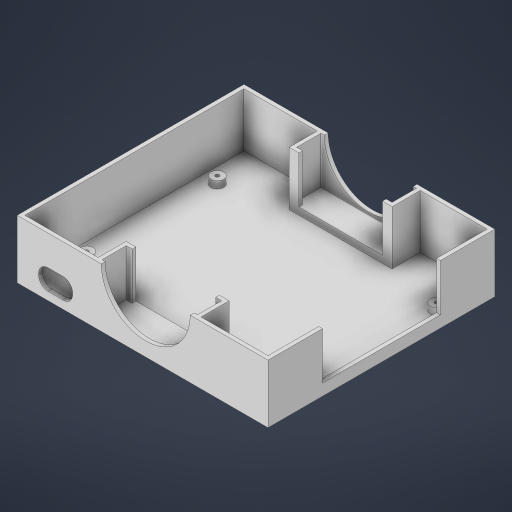
# Autodesk Inventor part: orangepicover-002
Saved by Autodesk Inventor 2023 (Build 270158000, 158)
## iProperties
Created: 2024-02-19
Part Number: orangepicover-002
Material: Generic
Document SubType Name: Modeling
Designer: Paul
Density: 1 g/cm^3
Appearance: Default
Author: Paul
Autodesk Inventor part; units mm, degrees
ref_plane "Work Plane1" through (0, 0, 0) normal (0, 0, 1) x (1, 0, 0)
sketch "Sketch1" plane through (0, 0, 0) normal (0, 0, 1) x (1, 0, 0)
  line L0 (-51.7982, 21.731) -> (-51.7982, 11.231) projected
  line L1 (-52.2736, -10.8209) -> (-52.2736, 4.8763)
  line L2 (4.6436, -33.7466) -> (19.655, -33.7466)
  line L3 (52.2917, 11.1414) -> (52.2917, 22.8908)
  line L4 (53.3077, -47.7466) -> (53.3077, 45.916)
  line L5 (-48.73, 30.9) -> (48.73, 30.9) projected
  line L6 (-52.2736, 31.916) -> (53.3077, 31.916) construction
  line L7 (-50.6226, 45.916) -> (53.3077, 45.916)
  line L8 (-50.6226, -47.7466) -> (53.3077, -47.7466)
  line L9 (-52.2736, 47.567) -> (-52.2736, -49.3976)
  line L10 (-50.6226, 45.916) -> (-50.6226, -47.7466)
  line L11 (54.9587, 47.567) -> (-52.2736, 47.567)
  line L12 (-52.2736, -49.3976) -> (54.9587, -49.3976)
  line L13 (54.9587, -49.3976) -> (54.9587, 47.567)
  point P0 (0, 0)
  dimension "d0" = 1.016
  dimension "d1" = 1.016
  dimension "d2" = 14
  dimension "d3" = 14
  dimension "d5" = 1.651
  dimension "d6" = 1.651
  dimension "d7" = 1.651
  dimension "d8" = 0
  dimension "d9" = 1.651
  constraints: 24 end point, 4 parallel, 2 point on line, 2 vertical, 1 horizontal, 6 other
  measures "d0" distance between parallel lines of L3 L4
  measures "d1" distance between parallel lines of L5 L6
  measures "d2" distance between parallel lines of L6 L7
  measures "d3" distance between parallel lines of L2 L8
  measures "d5" distance between parallel lines of L7 L11
  measures "d6" distance between parallel lines of L12 L8
  measures "d7" distance between parallel lines of L4 L13
  measures "d8" distance between parallel lines of L1 L9
  measures "d9" distance between parallel lines of L9 L10
extrude "Extrusion1" add sketch "Sketch1" against normal blind 20
sketch "Sketch2" plane through (0, 0, 0) normal (0, 0, 1) x (1, 0, 0)
  line L0 (-52.2736, 47.567) -> (-52.2736, -49.3976) projected
  line L1 (-52.2736, -49.3976) -> (54.9587, -49.3976) projected
  line L2 (54.9587, -49.3976) -> (54.9587, 47.567) projected
  line L3 (54.9587, 47.567) -> (-52.2736, 47.567) projected
  line L4 (-50.6226, 45.916) -> (53.3077, 45.916) projected
  line L5 (53.3077, 45.916) -> (53.3077, -47.7466) projected
  line L6 (53.3077, -47.7466) -> (-50.6226, -47.7466) projected
  line L7 (-50.6226, -47.7466) -> (-50.6226, 45.916) projected
  point P0 (0, 0)
extrude "Extrusion2" add sketch "Sketch2" along normal blind 5
sketch "Sketch3" plane through (0, 0, 5) normal (0, 0, 1) x (1, 0, 0)
  line L0 (-52.2736, 47.567) -> (-52.2736, -49.3976) projected
  line L1 (54.9587, 47.567) -> (-52.2736, 47.567) projected
  line L2 (54.9587, -49.3976) -> (54.9587, 47.567) projected
  line L3 (-52.2736, -49.3976) -> (54.9587, -49.3976) projected
  point P0 (0, 0)
extrude "Extrusion3" add sketch "Sketch3" against normal blind 2
sketch "Sketch4" plane through (0, 0, 3) normal (0, 0, -1) x (-1, 0, 0)
  circle A0 centre (47.0077, 28.0411) radius 1.45 construction
  circle A1 centre (-46.8473, 28.0411) radius 1.45 construction
  circle A2 centre (-46.8473, -27.8489) radius 1.45 construction
  circle A3 centre (47.0077, -27.8489) radius 1.45 construction
  circle A4 centre (47.0077, -27.8489) radius 2.72
  circle A5 centre (-46.8473, -27.8489) radius 2.72
  circle A6 centre (-46.8473, 28.0411) radius 2.72
  circle A7 centre (47.0077, 28.0411) radius 2.72
  point P0 (0, 0)
  dimension "d16" = 1.27
  constraints: 4 centre point, 3 equal radius
  measures "d16" radial gap between concentric circles of A3 A4
extrude "Extrusion4" add sketch "Sketch4" along normal blind 3
sketch "Sketch5" plane through (-52.2736, -49.3976, -20) normal (-1, 0, 0) x (0, 0, 1)
  line L0 (17.7, 27.0811) -> (5.5, 27.0811) projected
  line L1 (2.6, 71.1286) -> (2.6, 60.6286) projected
  line L2 (4.16, 72.4286) -> (8.16, 72.4286) projected
  line L3 (18.8, 72.9298) -> (18.8, 19.7676)
  line L4 (18.8, 27.0811) -> (2.6, 27.0811) construction
  line L5 (2.6, 27.0811) -> (2.6, 72.4287) construction
  line L6 (2.6, 72.4287) -> (18.8, 72.4287) construction
  line L7 (18.8, 72.4287) -> (18.8, 27.0811) construction
  line L8 (20.07, 23.2711) -> (20.07, 73.6987)
  line L9 (20.07, 73.6987) -> (0, 73.6987)
  line L10 (20.07, 23.2711) -> (0, 23.2711)
  line L11 (0, 96.9646) -> (0, 73.6935) projected
  line L12 (0, 0) -> (0, 96.9646) projected
  point P0 (20, 49.3976)
  dimension "d19" = 16.2
  dimension "d28" = 45.3475
  dimension "d29" = 1.27
  dimension "d30" = 3.81
  dimension "d31" = 1.27
  constraints: 16 end point, 4 point on line, 2 parallel, 1 horizontal, 1 perpendicular, 1 vertical, 2 other
  measures "d19" distance of L4.start L4.end
  measures "d28" distance of L4.end L5.end
  measures "d29" distance between parallel lines of L9 L2
  measures "d30" distance between parallel lines of L10 L0
  measures "d31" distance between parallel lines of L8 L7
extrude "Extrusion5" cut sketch "Sketch5" against normal blind 3
sketch "Sketch6" plane through (-52.2736, -49.3976, -20) normal (0, -1, 0) x (1, 0, 0)
  spline S0 degree 3 poles (96.7423, 17.4713) (96.7421, 17.4836) (96.7307, 17.9286) (96.5147, 18.8754) (95.3569, 20.0332) (94.4077, 20.2413) (93.9636, 20.25) knots 0 0 0 0 0.009266 0.335677 0.66431 1 1 1 1 construction
  line L0 (93.9636, 20.25) -> (87.581, 20.25) construction
  spline S1 degree 3 poles (87.581, 20.25) (87.5687, 20.2498) (87.1237, 20.2384) (86.1769, 20.0224) (85.0191, 18.8646) (84.811, 17.9154) (84.8023, 17.4713) knots 0 0 0 0 0.009266 0.335677 0.66431 1 1 1 1 construction
  line L1 (84.8023, 17.4713) -> (84.8023, 16.8687) construction
  spline S2 degree 3 poles (84.8023, 16.8687) (84.8025, 16.8564) (84.8139, 16.4114) (85.0299, 15.4646) (86.1877, 14.3068) (87.1369, 14.0987) (87.581, 14.09) knots 0 0 0 0 0.009266 0.335677 0.66431 1 1 1 1 construction
  line L2 (87.581, 14.09) -> (93.9636, 14.09) construction
  spline S3 degree 3 poles (93.9636, 14.09) (93.9759, 14.0902) (94.4209, 14.1016) (95.3677, 14.3176) (96.5255, 15.4754) (96.7336, 16.4246) (96.7423, 16.8687) knots 0 0 0 0 0.009266 0.335677 0.66431 1 1 1 1 construction
  line L3 (96.7423, 16.8687) -> (96.7423, 17.4713) construction
  circle A0 centre (90.7723, 17.17) radius 2.5 construction
  line L4 (93.9884, 12.82) -> (87.5562, 12.82)
  line L5 (83.5323, 16.8439) -> (83.5323, 17.4961)
  line L6 (87.5562, 21.52) -> (93.9884, 21.52)
  line L7 (98.0123, 17.4961) -> (98.0123, 16.8439)
  spline S4 degree 4 poles (87.5562, 12.8202) (87.0451, 12.8307) (86.5365, 12.9185) (85.5165, 13.2808) (84.696, 13.9837) (83.9931, 14.8042) (83.6308, 15.8242) (83.543, 16.3328) (83.5325, 16.8439) knots 0 0 0 0 0 0.32448 0.32448 0.675511 0.675511 1 1 1 1 1
  spline S5 degree 4 poles (83.5325, 17.4961) (83.5431, 18.0072) (83.6308, 18.5158) (83.9931, 19.5358) (84.696, 20.3563) (85.5165, 21.0592) (86.5365, 21.4215) (87.0451, 21.5092) (87.5562, 21.5198) knots 0 0 0 0 0 0.32448 0.32448 0.675511 0.675511 1 1 1 1 1
  spline S6 degree 4 poles (93.9884, 21.5198) (94.4995, 21.5092) (95.0081, 21.4215) (96.0281, 21.0592) (96.8486, 20.3563) (97.5515, 19.5358) (97.9138, 18.5158) (98.0016, 18.0072) (98.0121, 17.4961) knots 0 0 0 0 0 0.32448 0.32448 0.675511 0.675511 1 1 1 1 1
  spline S7 degree 4 poles (98.0121, 16.8439) (98.0015, 16.3328) (97.9138, 15.8242) (97.5515, 14.8042) (96.8486, 13.9837) (96.0281, 13.2808) (95.0081, 12.9185) (94.4995, 12.8307) (93.9884, 12.8202) knots 0 0 0 0 0 0.32448 0.32448 0.675511 0.675511 1 1 1 1 1
  point P0 (52.2736, 20)
  dimension "d24" = 1.27
  constraints: 8 end point, 7 parallel, 12 other
  measures "d24" distance between parallel lines of L2 L4
extrude "Extrusion6" cut sketch "Sketch6" against normal blind 3
sketch "Sketch7" plane through (0, 0, 3) normal (0, 0, -1) x (-1, 0, 0)
  line L0 (50.6226, -47.7466) -> (-53.3077, -47.7466) projected
  line L1 (0, -68.7905) -> (0, 66.9599) projected
  line L2 (50.6226, -47.7466) -> (-53.3077, -47.7466) projected
  line L3 (-22, -47.7466) -> (22, -47.7466)
  line L4 (22, -47.7466) -> (22, -35.7466)
  line L5 (22, -35.7466) -> (-22, -35.7466)
  line L6 (-22, -35.7466) -> (-22, -47.7466)
  point P0 (0, 0)
  point P1 (22, -47.7466)
  dimension "d32" = 44
  dimension "d33" = 22
  dimension "d34" = 12
  constraints: 8 end point, 2 parallel, 1 horizontal, 1 perpendicular, 1 point on line
  measures "d32" distance of L4.end L5.end
  measures "d33" distance between parallel lines of L6 L1
  measures "d34" distance of L3.end L4.end
ref_plane "Work Plane2" through (-18.0279, -47.6958, 0.0279) normal (0, 0, 1) x (1, 0, 0)
extrude "Extrusion7" add sketch "Sketch7" along normal up to surface (2.9721 mm away)
sketch "Sketch8" plane through (22, -35.7466, 0.0279) normal (0, 0, -1) x (-1, 0, 0)
  line L0 (44, 0) -> (0, 0) projected
  line L1 (0, 0) -> (0, -12) projected
  line L2 (44, -12) -> (0, -12) construction
  line L3 (44, -12) -> (44, 0) projected
  line L4 (42.4, -1.6) -> (42.4, -12)
  line L5 (1.6, -12) -> (1.6, -1.6)
  line L6 (4.14, 0) -> (4.14, -1.6)
  line L7 (1.6, -1.6) -> (4.14, -1.6)
  line L8 (39.86, -1.6) -> (42.4, -1.6)
  line L9 (0, -12) -> (1.6, -12)
  line L10 (42.4, -12) -> (44, -12)
  line L11 (39.86, -1.6) -> (39.86, 0)
  point P0 (22, 35.7466)
  point P1 (4.14, -0.8)
  dimension "d47" = 2.54
  dimension "d48" = 2.54
  dimension "d49" = 1.6
  dimension "d50" = 1.6
  dimension "d51" = 1.6
  dimension "d52" = 1.6
  constraints: 16 end point, 4 point on line, 3 perpendicular, 2 collinear, 1 midpoint
  measures "d47" distance from line of L5 point (4.14, -0.8)
  measures "d48" distance between parallel lines of L4 L11
  measures "d49" distance between parallel lines of L1 L5
  measures "d50" distance between parallel lines of L0 L7
  measures "d51" distance between parallel lines of L3 L4
  measures "d52" distance between parallel lines of L0 L8
extrude "Extrusion8" add sketch "Sketch8" along normal up to surface (20.0279 mm away)
sketch "Sketch9" plane through (-52.2736, -49.3976, -20) normal (0, -1, 0) x (1, 0, 0)
  line L0 (52.2736, 30) -> (52.2736, -5) projected
  line L1 (107.2323, 0) -> (0, 0) projected
  arc A0 (71.2736, 0) -> (33.2736, 0) centre (52.2736, 0) ccw
  point P0 (52.2736, 20)
  dimension "d53" = 38
  constraints: 4 point on line, 2 point on circle, 1 centre point
  measures "d53" diameter of A0
extrude "Extrusion9" cut sketch "Sketch9" against normal up to surface (1.651 mm away)
sketch "Sketch10" plane through (0, 0, 3) normal (0, 0, -1) x (-1, 0, 0)
  line L0 (0, -68.7905) -> (0, 66.9599) construction
  line L1 (-53.3077, 45.916) -> (50.6226, 45.916) construction
  line L2 (22, 45.916) -> (-22, 45.916)
  line L3 (-22, 45.916) -> (-22, 33.916)
  line L4 (-22, 33.916) -> (22, 33.916)
  line L5 (22, 33.916) -> (22, 45.916)
  point P0 (0, 0)
  dimension "d56" = 12
  dimension "d57" = 44
  dimension "d58" = 22
  constraints: 8 end point, 2 parallel, 1 horizontal, 1 perpendicular, 1 point on line
  measures "d56" distance of L4.end L2.start
  measures "d57" distance of L3.end L4.end
  measures "d58" distance between parallel lines of L5 L0
ref_plane "Work Plane3" through (-18.0279, 34.4686, 0.0279) normal (0, 0, 1) x (1, 0, 0)
extrude "Extrusion10" add sketch "Sketch10" along normal up to surface (2.9721 mm away)
sketch "Sketch11" plane through (22, 45.916, 0.0279) normal (0, 0, -1) x (-1, 0, 0)
  line L0 (44, -12) -> (0, -12) projected
  line L1 (44, 0) -> (44, -12) projected
  line L2 (0, -12) -> (0, 0) projected
  line L3 (-31.3077, 0) -> (72.6226, 0) construction
  line L4 (1.6, 0) -> (1.6, -10.4)
  line L5 (42.4, -10.4) -> (42.4, 0)
  line L6 (0, -12) -> (44, -12) projected
  line L7 (39.86, -12) -> (39.86, -10.4)
  line L8 (4.14, -12) -> (4.14, -10.4)
  line L9 (44, 0) -> (42.4, 0)
  line L10 (1.6, 0) -> (0, 0)
  line L11 (1.6, -10.4) -> (4.14, -10.4)
  line L12 (39.86, -10.4) -> (42.4, -10.4)
  point P0 (22, -45.916)
  point P1 (4.14, -12)
  point P2 (39.86, -12)
  dimension "d62" = 1.6
  dimension "d63" = 2.54
  dimension "d64" = 1.6
  dimension "d65" = 1.6
  dimension "d66" = 1.6
  dimension "d67" = 2.54
  constraints: 16 end point, 4 perpendicular, 2 point on line, 1 collinear, 1 horizontal
  measures "d62" distance between parallel lines of L1 L5
  measures "d63" distance between parallel lines of L5 L7
  measures "d64" distance between parallel lines of L0 L12
  measures "d65" distance between parallel lines of L0 L11
  measures "d66" distance between parallel lines of L2 L4
  measures "d67" distance between parallel lines of L4 L8
extrude "Extrusion11" add sketch "Sketch11" along normal up to surface (20.0279 mm away)
sketch "Sketch12" plane through (-52.2736, 47.567, -20) normal (0, 1, 0) x (1, 0, 0)
  line L0 (52.2736, 5) -> (52.2736, -30) construction
  line L1 (0, 0) -> (107.2323, 0) projected
  line L2 (72.6736, 0) -> (31.8736, 0) projected
  arc A0 (33.2736, 0) -> (71.2736, 0) centre (52.2736, 0) ccw
  point P0 (52.2736, -20)
  point P1 (71.2736, 0)
  point P2 (33.2736, 0)
  dimension "d70" = 38
  constraints: 2 point on circle, 2 point on line, 1 centre point, 1 midpoint
  measures "d70" diameter of A0
extrude "Extrusion12" cut sketch "Sketch12" against normal up to surface (1.651 mm away)
sketch "Sketch13" plane through (46.8473, 28.0411, 0) normal (0, 0, -1) x (-1, 0, 0)
  circle A0 centre (0, -55.89) radius 2.72 projected
  circle A1 centre (0, 0) radius 2.72 projected
  circle A2 centre (93.855, 0) radius 2.72 projected
  circle A3 centre (93.855, -55.89) radius 2.72 projected
  point P0 (46.8473, -28.0411)
  constraints: 4 coincident
hole "Hole1" at (46.8473, -27.8489, 0) at (46.8473, 28.0411, 0) at (-47.0077, 28.0411, 0) at (-47.0077, -27.8489, 0) direction (0, 0, 1) diameter 1.567 end through all thread size "M2x0.4" class "6H" standard "ANSI Metric M Profile"
equation "\"d33\" = 0.5 * d32"
equation "\"d48\" = d47"
equation "\"d50\" = d49"
equation "\"d51\" = d49"
equation "\"d52\" = d49"
equation "\"d58\" = 0.5 * d57"
equation "\"d64\" = d62"
equation "\"d65\" = d62"
equation "\"d66\" = d62"
equation "\"d67\" = d63"
body "Solid1"
